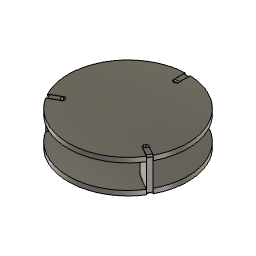
Blinkies-TDOW-Freilab v3 (Autodesk Fusion 360 design; units mm, degrees)
Autodesk Fusion 360 part; units mm, degrees
note: some values were not read from the file. Set by a fixed rule: which sketch regions a step uses.
sketch "Base Sketch" plane through (0, 0, 0) normal (0, 0, 1) x (1, 0, 0)
  line L0 (0.85, 19.9819) -> (0.85, 15.9819)
  line L1 (0.25, 15.3819) -> (-0.25, 15.3819)
  line L2 (-0.85, 15.9819) -> (-0.85, 19.9819)
  line L3 (0, 1.75) -> (0, 22.5)
  arc A0 (-0.85, 15.9819) -> (-0.25, 15.3819) centre (-0.25, 15.9819) ccw
  arc A1 (0.25, 15.3819) -> (0.85, 15.9819) centre (0.25, 15.9819) ccw
  line L4 (-13.4158, -8.7271) -> (-16.8799, -10.7271)
  arc A2 (-13.4158, -8.7271) -> (-13.1961, -7.9075) centre (-13.7158, -8.2075) ccw
  line L5 (-13.4461, -7.4745) -> (-13.1961, -7.9075)
  arc A3 (-13.4461, -7.4745) -> (-14.2658, -7.2548) centre (-13.9658, -7.7745) ccw
  line L6 (-17.7299, -9.2548) -> (-14.2658, -7.2548)
  line L7 (14.2658, -7.2548) -> (17.7299, -9.2548)
  arc A4 (14.2658, -7.2548) -> (13.4461, -7.4745) centre (13.9658, -7.7745) ccw
  line L8 (13.1961, -7.9075) -> (13.4461, -7.4745)
  arc A5 (13.1961, -7.9075) -> (13.4158, -8.7271) centre (13.7158, -8.2075) ccw
  line L9 (16.8799, -10.7271) -> (13.4158, -8.7271)
  arc A6 (17.7299, -9.2548) -> (0.85, 19.9819) centre (0, 0) ccw
  arc A7 (-16.8799, -10.7271) -> (16.8799, -10.7271) centre (0, 0) ccw
  arc A8 (17.7299, -9.2548) -> (0.85, 19.9819) centre (0, 0) ccw
  arc A9 (-0.85, 19.9819) -> (-17.7299, -9.2548) centre (0, 0) ccw
  point P0 (-0.85, 15.3819)
  dimension "d1" = 40
  dimension "d6" = 1.7
  dimension "d7" = 4.6
  dimension "d8" = 0.6
  dimension "d10" = 360
  constraint coincident A6.centre A7.centre
  constraint vertical L0
  constraint horizontal L1
  constraint vertical L2
  constraint symmetric L0 L2 L3
  constraint coincident P0 L1
  constraint coincident P0 L2
  constraint tangent L1 A0
  constraint tangent L2 A0
  constraint tangent L0 A1
  constraint tangent L1 A1
  constraint equal A0 A1
  constraint concentric A6 A7
  constraint concentric A7 A8
  constraint concentric A8 A9
  measures "d1" diameter of A7
  measures "d6" distance of L2.end L0.start
  measures "d7" distance of L2.end P0
  measures "d8" radius of A0
extrude "Extrude1" add sketch "Base Sketch" along normal blind 1.6 makes body 1
sketch "Tab Sketch" plane through (0, 0, 0) normal (1, 0, 0) x (0, 1, 0)
  line L0 (15.9819, 0) -> (19.9819, 0)
  line L1 (19.9819, 0) -> (19.9819, 1.6)
  line L2 (19.9819, 1.6) -> (15.9819, 1.6)
  line L3 (15.9819, 1.6) -> (15.9819, 0)
  line L4 (15.9819, 1.6) -> (14.4819, 1.6)
  line L5 (13.9819, 2.1) -> (13.9819, 9.1)
  line L6 (14.4819, 9.6) -> (15.9819, 9.6)
  line L7 (19.9819, 9.6) -> (19.9819, 1.6)
  line L8 (15.9819, 9.6) -> (15.9819, 10.7)
  line L9 (16.4819, 11.2) -> (19.4819, 11.2)
  line L10 (19.9819, 10.7) -> (19.9819, 9.6)
  line L11 (19.9819, 1.6) -> (19.9819, 0.5)
  line L12 (19.4819, 0) -> (16.4819, 0)
  line L13 (15.9819, 0.5) -> (15.9819, 1.6)
  arc A0 (19.4819, 0) -> (19.9819, 0.5) centre (19.4819, 0.5) ccw
  arc A1 (15.9819, 0.5) -> (16.4819, 0) centre (16.4819, 0.5) ccw
  arc A2 (13.9819, 2.1) -> (14.4819, 1.6) centre (14.4819, 2.1) ccw
  arc A3 (14.4819, 9.6) -> (13.9819, 9.1) centre (14.4819, 9.1) ccw
  arc A4 (16.4819, 11.2) -> (15.9819, 10.7) centre (16.4819, 10.7) ccw
  arc A5 (19.9819, 10.7) -> (19.4819, 11.2) centre (19.4819, 10.7) ccw
  point P0 (13.9819, 1.6)
  point P1 (19.9819, 11.2)
  point P2 (15.9819, 0)
  dimension "d13" = 6
  dimension "d14" = 8
  dimension "d15" = 4
  dimension "d16" = 1.6
  dimension "d17" = 4
  dimension "d18" = 1.6
  dimension "d19" = 0.5
  constraint horizontal L4
  constraint vertical L5
  constraint horizontal L6
  constraint vertical L7
  constraint coincident L1.end L2.start
  constraint vertical L8
  constraint horizontal L9
  constraint vertical L10
  constraint vertical L11
  constraint horizontal L12
  constraint vertical L13
  constraint coincident L2.end L3.start
  constraint tangent L11 A0
  constraint tangent L12 A0
  constraint coincident P2 L12
  constraint coincident P2 L13
  constraint tangent L12 A1
  constraint tangent L13 A1
  constraint equal A0 A1
  constraint coincident P0 L4
  constraint coincident P0 L5
  constraint tangent L4 A2
  constraint tangent L5 A2
  constraint equal A0 A2
  constraint tangent L5 A3
  constraint tangent L6 A3
  constraint equal A0 A3
  constraint tangent L8 A4
  constraint tangent L9 A4
  constraint equal A0 A4
  constraint coincident P1 L9
  constraint coincident P1 L10
  constraint tangent L9 A5
  constraint tangent L10 A5
  constraint equal A0 A5
  constraint horizontal L7.start L6.end
  measures "d13" distance of L1.end P0
  measures "d14" distance of L1.end L7.start
  measures "d15" distance of L7.start L6.end
  measures "d16" distance of L7.start P1
  measures "d17" distance of L2.end L1.end
  measures "d18" distance of L2.end P2
  measures "d19" radius of A0
extrude "Extrude2" add sketch "Tab Sketch" along normal mid plane 1.6 separate body contours L0 L1 L2 L3 L11 L12 L13 A0 A1 | L2 L4 L5 L6 L7 L8 L9 L10 A2 A3 A4 A5 makes body 2
pattern_circular "C-Pattern1" count 3 over 360 about axis through (0, 0, 1.6) along (0, 0, 1) of bodies 2 makes body 3 at (-15.7502, -10.0171, 6.9333) makes body 4 at (16.5502, -8.6315, 6.9333)
ref_plane "WorkPlane1" through (0, 17.9819, 5.6) normal (0, 0, 1) x (0, -1, 0)
mirror "Mirror1" about plane through (0, 17.9819, 5.6) normal (0, 0, 1) of bodies 1 makes body 5
equation "tab_depth = 4 mm"
equation "pcb_thickness = 1.6 mm"
equation "slot_radius = 0.6 mm"
equation "slot_tolerance = 0.1 mm"
equation "d6 = pcb_thickness + slot_tolerance"
equation "d7 = tab_depth + slot_radius"
equation "d8 = slot_radius"
equation "d11 = pcb_thickness"
equation "d15 = tab_depth"
equation "d16 = pcb_thickness"
equation "d17 = tab_depth"
equation "d18 = pcb_thickness"
equation "d20 = pcb_thickness"
named bodies: "Base", "Tab", "Tab (1)", "Tab (2)", "Base (1)"
